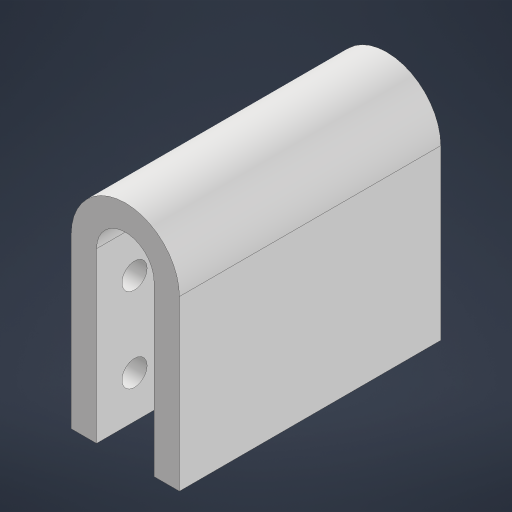
# Autodesk Inventor part: back_helmet_holder
Saved by Autodesk Inventor 2024 (Build 280153000, 153)
## iProperties
Created: 2026-08-20
Part Number: back_helmet_holder
Material: Generic
Document SubType Name: Modeling
Designer: schar
Density: 1 g/cm^3
Appearance: Default
Author: schar
Autodesk Inventor part; units mm, degrees
ref_plane "YZ Plane" through (0, 0, 0) normal (1, 0, 0) x (0, 1, 0)
ref_plane "XZ Plane" through (0, 0, 0) normal (0, 1, 0) x (-1, 0, 0)
ref_plane "XY Plane" through (0, 0, 0) normal (0, 0, 1) x (1, 0, 0)
sketch "Sketch1" plane through (0, 0, 0) normal (0, 0, 1) x (1, 0, 0)
  line L0 (0, 20) -> (0, 0) projected
  line L1 (0, 20) -> (-3, 20) projected
  line L2 (-3, 0) -> (-3, 20) projected
  line L3 (0, 0) -> (-3, 0) projected
  arc A0 (-3, 20) -> (-9.8284, 20) centre (-6.4142, 20) ccw
  circle A1 centre (-6.4142, 20) radius 6.4142
  line L4 (-9.8284, 20) -> (-12.8284, 20)
  line L5 (-12.8284, 20) -> (-12.8284, 0)
  line L6 (-12.8284, 0) -> (-9.8284, 0)
  line L7 (-9.8284, 0) -> (-9.8284, 20)
  point P0 (-3, 14.57)
  constraints: 8 end point, 2 parallel, 2 point on circle, 1 centre point, 1 coincident, 1 horizontal, 1 perpendicular, 1 point on line, 1 tangent, 3 other
ref_plane "Work Plane1" through (-3, 0, 31) normal (0, 0, -1) x (0, 1, 0)
extrude "Extrusion1" add sketch "Sketch1" along normal up to surface (31 mm away) contours A1 L2 L1 | L1 A0 L4 A1 | L0 L3 L2 A1 | L4 L7 A1 | A1 L7 L6 L5
sketch "Sketch2" plane through (-12.8284, 0, 0) normal (-1, 0, 0) x (0, 0, 1)
  line L0 (0, 0) -> (31, 0) projected
  line L1 (15.5, 0) -> (15.5, 20)
  line L2 (0, 20) -> (31, 20) projected
  line L3 (15.5, 10) -> (4.5, 10)
  line L4 (15.5, 10) -> (26.5, 10)
  line L5 (26.5, 10) -> (26.5, 5)
  line L6 (4.5, 10) -> (4.5, 15)
  circle A0 centre (26.5, 5) radius 1.5
  circle A1 centre (4.5, 15) radius 1.5
  line L7 (26.5, 5) -> (4.5, 5)
  line L8 (4.5, 5) -> (4.5, 15)
  line L9 (4.5, 15) -> (26.5, 15)
  line L10 (26.5, 15) -> (26.5, 5)
  circle A2 centre (4.5, 5) radius 1.5
  circle A3 centre (26.5, 15) radius 1.5
  dimension "d2" = 11
  dimension "d3" = 11
  dimension "d4" = 5
  dimension "d5" = 5
  dimension "d6" = 3
  dimension "d7" = 3
  dimension "d8" = 3
  dimension "d9" = 3
  constraints: 18 end point, 4 centre point, 4 coincident, 3 horizontal, 3 midpoint, 2 parallel, 2 vertical, 1 perpendicular
  measures "d2" distance of L3.start L3.end
  measures "d3" distance of L3.start L4.end
  measures "d4" distance of L4.end L5.end
  measures "d5" distance of L3.end L6.end
  measures "d6" diameter of A0
  measures "d7" diameter of A1
  measures "d8" diameter of A2
  measures "d9" diameter of A3
extrude "Extrusion2" cut sketch "Sketch2" against normal up to surface (3 mm away) contours L7 L5 A0 | A0 L5 L7 | A2 L8 L7 | L7 L8 A2 | L9 L6 A1 | A1 L6 L9 | A3 L10 L9 | L9 L10 A3
body "Solid1"
